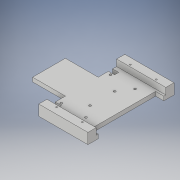
# Autodesk Inventor part: MotorPlate
Saved by Autodesk Inventor 2019 (Build 230136000, 136)
## iProperties
Created: 2019-10-06
Part Number: MotorPlate
Material: Generic
Document SubType Name: Modeling
Designer: james
Density: 1 g/cm^3
Appearance: Default
Author: james
Autodesk Inventor part; units mm, degrees
ref_plane "YZ Plane" through (0, 0, 0) normal (1, 0, 0) x (0, 1, 0)
ref_plane "XZ Plane" through (0, 0, 0) normal (0, 1, 0) x (-1, 0, 0)
ref_plane "XY Plane" through (0, 0, 0) normal (0, 0, 1) x (1, 0, 0)
sketch "Sketch1" plane through (0, 0, 0) normal (0, 1, 0) x (-1, 0, 0)
  line L0 (103.6935, 180.0499) -> (-48.7065, 180.0499)
  line L1 (-48.7065, 180.0499) -> (-48.7065, -86.6501)
  line L2 (-48.7065, -86.6501) -> (103.6935, -86.6501)
  line L3 (103.6935, -86.6501) -> (103.6935, 180.0499)
  point P0 (0, 0)
  dimension "d0" = 266.7
  dimension "d1" = 152.4
  constraints: 8 end point, 2 parallel, 1 horizontal, 1 perpendicular
  measures "d0" distance of L0.end L1.end
  measures "d1" distance of L0.start L0.end
extrude "Extrusion1" add sketch "Sketch1" along normal blind 12.7
sketch "Sketch2" plane through (0, 12.7, 0) normal (0, 1, 0) x (1, 0, 0)
  line L0 (-103.6935, 86.6501) -> (-103.6935, -180.0499) projected
  line L1 (-103.6935, -180.0499) -> (48.7065, -180.0499)
  line L2 (48.7065, -180.0499) -> (48.7065, -154.6499)
  line L3 (48.7065, -154.6499) -> (-103.6935, -154.6499)
  line L4 (-103.6935, -154.6499) -> (-103.6935, -180.0499)
  line L5 (48.7065, -180.0499) -> (48.7065, 86.6501) projected
  line L6 (48.7065, 86.6501) -> (-103.6935, 86.6501)
  line L7 (-103.6935, 86.6501) -> (-103.6935, 61.2501)
  line L8 (-103.6935, 61.2501) -> (48.7065, 61.2501)
  line L9 (48.7065, 61.2501) -> (48.7065, 86.6501)
  point P0 (0, 0)
  dimension "d4" = 25.4
  dimension "d5" = 25.4
  dimension "d8" = 0
  constraints: 16 end point, 4 parallel, 2 horizontal, 2 perpendicular, 1 point on line
  measures "d4" distance between parallel lines of L6 L8
  measures "d5" distance between parallel lines of L1 L3
  measures "d8" distance between parallel lines of L2 L5
extrude "Extrusion2" add sketch "Sketch2" along normal blind 20.1422 contours L6 L5 L8 L0 | L3 L2 L1 L0
sketch "Sketch3" plane through (0, 0, 0) normal (0, -1, 0) x (1, 0, 0)
  line L0 (94.7395, 46.6999) -> (-172.7542, 46.6999)
  line L1 (-103.6935, 180.0499) -> (48.7065, 180.0499) projected
  line L2 (-27.4935, 259.5672) -> (-27.4935, -153.6047)
  line L3 (48.7065, 180.0499) -> (48.7065, -86.6501) projected
  point P0 (0, 0)
  point P1 (12.5115, 160.9999)
  point P2 (-67.4985, 160.9999)
  point P3 (12.5115, -67.6001)
  point P4 (-67.4985, -67.6001)
  dimension "d9" = 133.35
  dimension "d10" = 76.2
  dimension "d11" = 40.005
  dimension "d12" = 40.005
  dimension "d13" = 0
  dimension "d14" = 0
  dimension "d15" = 114.3
  dimension "d16" = 0
  dimension "d17" = 0
  dimension "d18" = 114.3
  constraints: 4 end point, 1 horizontal, 1 vertical
  measures "d9" distance between parallel lines of L1 L0
  measures "d10" distance between parallel lines of L2 L3
  measures "d11" distance from line of L2 point (12.511, 161)
  measures "d12" distance from line of point (-67.499, 161) L2
  measures "d13" horizontal distance of point (-67.499, -67.6) point (-67.499, 161)
  measures "d14" horizontal distance of point (12.511, 161) point (12.511, -67.6)
  measures "d15" distance from line of L0 point (12.511, 161)
  measures "d16" vertical distance of point (12.511, 161) point (-67.499, 161)
  measures "d17" vertical distance of point (-67.499, -67.6) point (12.511, -67.6)
  measures "d18" distance from line of L0 point (-67.499, -67.6)
hole "Hole1" at (12.5115, 0, 160.9999) at (-67.4985, 0, 160.9999) at (12.5115, 0, -67.6001) at (-67.4985, 0, -67.6001) direction (0, 1, 0) diameter 4.4958 end through all counterbore diameter 7.9502 counterbore depth 4.1656 clearance for "Socket Head Cap Screw" size "#8" standard "Ansi Unified Screw Threads"
sketch "Sketch4" plane through (-103.6935, 0, -86.6501) normal (-1, 0, 0) x (0, 0, 1)
  line L0 (184.15, 0) -> (82.55, 0)
  line L1 (82.55, 0) -> (82.55, 12.7)
  line L2 (82.55, 12.7) -> (184.15, 12.7)
  line L3 (184.15, 12.7) -> (184.15, 0)
  line L4 (0, 0) -> (0, 32.8422) projected
  line L5 (0, 0) -> (266.7, 0) projected
  line L6 (25.4, 12.7) -> (241.3, 12.7) projected
  line L7 (266.7, 0) -> (266.7, 32.8422) projected
  point P0 (86.6501, 0)
  dimension "d26" = 101.6
  dimension "d27" = 82.55
  dimension "d28" = 0
  dimension "d29" = 0
  dimension "d53" = 82.55
  constraints: 8 end point, 2 parallel, 1 horizontal, 1 perpendicular
  measures "d26" distance of L0.start L0.end
  measures "d27" distance between parallel lines of L4 L1
  measures "d28" distance between parallel lines of L5 L0
  measures "d29" distance between parallel lines of L6 L2
  measures "d53" distance between parallel lines of L7 L3
extrude "Extrusion3" add sketch "Sketch4" along normal blind 101.6
sketch "Sketch5" plane through (0, 0, 0) normal (0, -1, 0) x (1, 0, 0)
  line L0 (-103.6935, 97.4999) -> (-205.2935, 97.4999) projected
  line L1 (-103.6935, -4.1001) -> (-205.2935, -4.1001) projected
  line L2 (48.7065, 180.0499) -> (48.7065, -86.6501) projected
  line L3 (-103.6935, -86.6501) -> (-103.6935, -4.1001) projected
  point P0 (0, 0)
  point P1 (-14.7935, 122.8999)
  point P2 (-90.9935, 122.8999)
  point P3 (-90.9935, -29.5001)
  point P4 (-14.7935, -29.5001)
  dimension "d32" = 0
  dimension "d33" = 0
  dimension "d34" = 25.4
  dimension "d35" = 25.4
  dimension "d36" = 0
  dimension "d38" = 12.7
  dimension "d52" = 76.2
  dimension "d54" = 0
  measures "d32" vertical distance of point (-14.794, -29.5) point (-90.994, -29.5)
  measures "d33" vertical distance of point (-14.794, 122.9) point (-90.994, 122.9)
  measures "d34" distance from line of L0 point (-14.794, 122.9)
  measures "d35" distance from line of point (-90.994, -29.5) L1
  measures "d36" horizontal distance of point (-14.794, -29.5) point (-14.794, 122.9)
  measures "d38" distance from line of L3 point (-90.994, -29.5)
  measures "d52" distance of point (-90.994, -29.5) point (-14.794, -29.5)
  measures "d54" horizontal distance of point (-90.994, 122.9) point (-90.994, -29.5)
hole "Hole2" at (-14.7935, 0, 122.8999) at (-90.9935, 0, 122.8999) at (-90.9935, 0, -29.5001) at (-14.7935, 0, -29.5001) direction (0, 1, 0) diameter 4.4958 end through all
sketch "Sketch6" plane through (0, 12.7, 0) normal (0, 1, 0) x (1, 0, 0)
  circle A0 centre (-90.9935, -122.8999) radius 2.2479 projected
  circle A1 centre (-14.7935, -122.8999) radius 2.2479 projected
  circle A2 centre (-14.7935, 29.5001) radius 2.2479 projected
  circle A3 centre (-90.9935, 29.5001) radius 2.2479 projected
  circle A4 centre (-90.9935, 29.5001) radius 2.2479 projected
  circle A5 centre (-90.9935, 29.5001) radius 3.3734
  circle A6 centre (-90.9935, -122.8999) radius 3.3734
  circle A7 centre (-14.7935, -122.8999) radius 3.3734
  circle A8 centre (-14.7935, 29.5001) radius 3.3734
  point P0 (0, 0)
  dimension "d46" = 6.7469
  dimension "d47" = 6.7469
  dimension "d48" = 6.7469
  dimension "d49" = 6.7469
  constraints: 4 centre point, 4 coincident
  measures "d46" diameter of A5
  measures "d47" diameter of A6
  measures "d48" diameter of A7
  measures "d49" diameter of A8
extrude "Extrusion4" cut sketch "Sketch6" against normal blind 9.525 contours A0 | A1 | A2 | A3 | A5 | A6 | A7 | A8
sketch "Sketch7" plane through (0, 0, 0) normal (0, -1, 0) x (1, 0, 0)
  line L0 (85.2483, 148.2999) -> (23.3065, 148.2999)
  line L1 (23.3065, 148.2999) -> (23.3065, -54.9001)
  line L2 (23.3065, -54.9001) -> (85.2483, -54.9001)
  line L3 (85.2483, -54.9001) -> (85.2483, 148.2999)
  line L4 (48.7065, -86.6501) -> (-103.6935, -86.6501) projected
  line L5 (-103.6935, 180.0499) -> (48.7065, 180.0499) projected
  line L6 (48.7065, 180.0499) -> (48.7065, -86.6501) projected
  point P0 (0, 0)
  dimension "d55" = 31.75
  dimension "d56" = 31.75
  dimension "d57" = 25.4
  constraints: 8 end point, 2 parallel, 1 horizontal, 1 perpendicular
  measures "d55" distance between parallel lines of L4 L2
  measures "d56" distance between parallel lines of L5 L0
  measures "d57" distance between parallel lines of L1 L6
extrude "Extrusion5" cut sketch "Sketch7" against normal blind 50.8
sketch "Sketch8" plane through (0, 0, 0) normal (0, -1, 0) x (1, 0, 0)
  line L0 (-111.6685, 129.2499) -> (-84.6435, 129.2499)
  line L1 (-84.6435, 129.2499) -> (-84.6435, 141.9499)
  line L2 (-84.6435, 141.9499) -> (-111.6685, 141.9499)
  line L3 (-111.6685, 141.9499) -> (-111.6685, 129.2499)
  line L4 (-115.7126, -48.5501) -> (-84.6435, -48.5501)
  line L5 (-84.6435, -48.5501) -> (-84.6435, -35.8501)
  line L6 (-84.6435, -35.8501) -> (-115.7126, -35.8501)
  line L7 (-115.7126, -35.8501) -> (-115.7126, -48.5501)
  line L8 (-103.6935, -86.6501) -> (-103.6935, -4.1001) projected
  line L9 (-103.6935, 97.4999) -> (-103.6935, 180.0499) projected
  point P0 (0, 0)
  point P1 (-103.6935, -61.2501)
  point P2 (-103.6935, 154.6499)
  dimension "d60" = 12.7
  dimension "d61" = 12.7
  dimension "d62" = 19.05
  dimension "d63" = 19.05
  dimension "d64" = 12.7
  dimension "d65" = 12.7
  constraints: 16 end point, 4 parallel, 2 horizontal, 2 perpendicular
  measures "d60" distance from line of L4 point (-103.694, -61.25)
  measures "d61" distance of L4.end L5.end
  measures "d62" distance between parallel lines of L8 L5
  measures "d63" distance between parallel lines of L9 L1
  measures "d64" distance from line of point (-103.694, 154.65) L2
  measures "d65" distance of L2.end L0.start
extrude "Extrusion6" cut sketch "Sketch8" against normal blind 50.8
sketch "Sketch9" plane through (0, 0, 0) normal (0, -1, 0) x (1, 0, 0)
  line L0 (-103.6935, 180.0499) -> (48.7065, 180.0499) projected
  line L1 (48.7065, 180.0499) -> (48.7065, 148.2999) projected
  point P0 (0, 0)
  point P1 (-40.1935, 84.7999)
  point P2 (-40.1935, 8.5999)
  dimension "d68" = 76.2
  dimension "d69" = 0
  dimension "d70" = 95.25
  dimension "d71" = 88.9
  measures "d68" distance of point (-40.194, 84.8) point (-40.194, 8.6)
  measures "d69" horizontal distance of point (-40.194, 84.8) point (-40.194, 8.6)
  measures "d70" distance from line of L0 point (-40.194, 84.8)
  measures "d71" distance from line of L1 point (-40.194, 8.6)
hole "Hole3" at (-40.1935, 0, 84.7999) at (-40.1935, 0, 8.5999) direction (0, 1, 0) diameter 4.4958 end through all clearance for "Flat Head Machine Screw (82)" size "#8" standard "Ansi Unified Screw Threads"
sketch "Sketch10" plane through (0, 12.7, 0) normal (0, 1, 0) x (1, 0, 0)
  circle A0 centre (-40.1935, -84.7999) radius 2.2479 projected
  circle A1 centre (-40.1935, -8.5999) radius 2.2479 projected
  circle A2 centre (-40.1935, -8.5999) radius 2.2479 projected
  circle A3 centre (-40.1935, -8.5999) radius 3.3734
  circle A4 centre (-40.1935, -84.7999) radius 3.3734
  point P0 (0, 0)
  dimension "d79" = 6.7469
  dimension "d80" = 6.7469
  constraints: 2 centre point, 2 coincident
  measures "d79" diameter of A4
  measures "d80" diameter of A3
extrude "Extrusion7" cut sketch "Sketch10" against normal blind 9.525 contours A0 | A1 | A3 | A4
body "Solid1"
